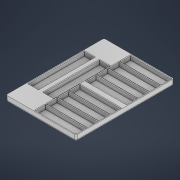
# Autodesk Inventor part: Pocker higher half
Saved by Autodesk Inventor 2022 (Build 260153000, 153)
## iProperties
Created: 2021-05-24
Part Number: Pocker higher half
Material: Aluminum 6061-AHC
Document SubType Name: Modeling
Designer: Albert L Tomberg
Density: 2.7 g/cm^3
Appearance: Aluminum - Polished
Author: Albert L Tomberg
Autodesk Inventor part; units mm, degrees
ref_plane "YZ Plane" through (0, 0, 0) normal (1, 0, 0) x (0, 1, 0)
ref_plane "XZ Plane" through (0, 0, 0) normal (0, 1, 0) x (-1, 0, 0)
ref_plane "XY Plane" through (0, 0, 0) normal (0, 0, 1) x (1, 0, 0)
sketch "Sketch1" plane through (0, 0, 0) normal (0, 1, 0) x (-1, 0, 0)
  line L0 (0, 0) -> (250, 0)
  line L1 (250, 0) -> (250, -350)
  line L2 (250, -350) -> (0, -350)
  line L3 (0, -350) -> (0, 0)
  dimension "d0" = 250
  dimension "d1" = 350
  constraints: 8 end point, 2 parallel, 1 horizontal, 1 perpendicular
  measures "d0" distance of L1.end L2.end
  measures "d1" distance of L0.end L1.end
extrude "Extrusion1" add sketch "Sketch1" along normal blind 20
sketch "Sketch2" plane through (0, 20, 0) normal (0, 1, 0) x (1, 0, 0)
  line L0 (-5, 5) -> (-150, 5)
  line L1 (-150, 5) -> (-150, 41)
  line L2 (-150, 41) -> (-5, 41)
  line L3 (-5, 41) -> (-5, 5)
  line L4 (-250, 0) -> (0, 0) projected
  line L5 (-250, 350) -> (-250, 0) projected
  line L6 (-150, 41) -> (-150, 46)
  line L7 (-150, 46) -> (-5, 46)
  line L8 (-5, 46) -> (-5, 82)
  line L9 (-5, 82) -> (-150, 82)
  line L10 (-150, 82) -> (-150, 46)
  line L11 (-150, 82) -> (-150, 87)
  line L12 (-150, 87) -> (-5, 87)
  line L13 (-5, 87) -> (-5, 123)
  line L14 (-5, 123) -> (-150, 123)
  line L15 (-150, 123) -> (-150, 87)
  line L16 (-150, 123) -> (-150, 128)
  line L17 (-150, 128) -> (-5, 128)
  line L18 (-5, 128) -> (-5, 164)
  line L19 (-5, 164) -> (-150, 164)
  line L20 (-150, 164) -> (-150, 128)
  line L21 (-5, 345) -> (-150, 345)
  line L22 (-150, 345) -> (-150, 309)
  line L23 (-150, 309) -> (-5, 309)
  line L24 (-5, 309) -> (-5, 345)
  line L25 (-5, 309) -> (-5, 304)
  line L26 (-5, 304) -> (-5, 268)
  line L27 (-5, 268) -> (-150, 268)
  line L28 (-150, 268) -> (-150, 304)
  line L29 (-150, 304) -> (-5, 304)
  line L30 (0, 0) -> (0, 350) projected
  line L31 (-150, 268) -> (-150, 263)
  line L32 (-150, 263) -> (-5, 263)
  line L33 (-5, 263) -> (-5, 227)
  line L34 (-5, 227) -> (-150, 227)
  line L35 (-150, 227) -> (-150, 263)
  line L36 (-5, 227) -> (-5, 222)
  line L37 (-5, 222) -> (-150, 222)
  line L38 (-150, 222) -> (-150, 186)
  line L39 (-150, 186) -> (-5, 186)
  line L40 (-5, 186) -> (-5, 222)
  line L41 (0, 350) -> (-250, 350) projected
  line L42 (-245, 75) -> (-245, 275)
  line L43 (-245, 275) -> (-209, 275)
  line L44 (-209, 275) -> (-209, 75)
  line L45 (-209, 75) -> (-245, 75)
  line L46 (-155, 75) -> (-155, 275)
  line L47 (-155, 275) -> (-191, 275)
  line L48 (-191, 275) -> (-191, 75)
  line L49 (-191, 75) -> (-155, 75)
  dimension "d4" = 145
  dimension "d5" = 36
  dimension "d6" = 5
  dimension "d7" = 100
  dimension "d8" = 5
  dimension "d9" = 36
  dimension "d10" = 5
  dimension "d11" = 36
  dimension "d12" = 5
  dimension "d13" = 36
  dimension "d14" = 36
  dimension "d15" = 5
  dimension "d16" = 36
  dimension "d17" = 5
  dimension "d18" = 36
  dimension "d19" = 5
  dimension "d20" = 36
  dimension "d21" = 5
  dimension "d22" = 5
  dimension "d23" = 5
  dimension "d24" = 200
  dimension "d25" = 36
  dimension "d26" = 36
  dimension "d27" = 5
  dimension "d28" = 75
  dimension "d29" = 18
  dimension "d30" = 75
  dimension "d31" = 75
  constraints: 92 end point, 25 perpendicular, 22 point on line, 6 parallel, 2 horizontal, 2 vertical
  measures "d4" distance of L1.end L2.end
  measures "d5" distance of L0.end L1.end
  measures "d6" distance between parallel lines of L4 L0
  measures "d7" distance between parallel lines of L5 L1
  measures "d8" distance of L1.end L6.end
  measures "d9" distance of L7.end L8.end
  measures "d10" distance of L9.end L11.end
  measures "d11" distance of L12.end L13.end
  measures "d12" distance of L14.end L16.end
  measures "d13" distance of L17.end L18.end
  measures "d14" distance of L21.end L22.end
  measures "d15" distance of L23.end L25.end
  measures "d16" distance of L25.end L26.end
  measures "d17" distance of L27.end L31.end
  measures "d18" distance of L32.end L33.end
  measures "d19" distance of L33.end L36.end
  measures "d20" distance of L37.end L38.end
  measures "d21" distance between parallel lines of L41 L21
  measures "d22" distance between parallel lines of L30 L8
  measures "d23" distance between parallel lines of L30 L13
  measures "d24" distance of L42.start L42.end
  measures "d25" distance of L42.end L43.end
  measures "d26" distance of L46.end L47.end
  measures "d27" distance between parallel lines of L5 L42
  measures "d28" distance between parallel lines of L4 L45
  measures "d29" distance between parallel lines of L44 L48
  measures "d30" distance between parallel lines of L4 L49
  measures "d31" distance between parallel lines of L41 L47
extrude "Extrusion2" cut sketch "Sketch2" against normal blind 15 contours L20 L19 L18 L17 | L15 L14 L13 L12 | L10 L9 L8 L7 | L0 L1 L2 L3 | L24 L23 L22 L21 | L40 L39 L38 L37 | L32 L33 L34 L35 | L26 L27 L28 L29 | L42 L43 L44 L45 | L49 L48 L47 L46
fillet "Fillet1" radius 5 8 edges at (-125, 0, 0) (0, 10, 0) (0, 0, -175) (0, 10, -350) (-125, 0, -350) (-250, 10, -350) (-250, 0, -175) (-250, 10, 0)
fillet "Fillet2" radius 1 79 edges at (-150, 5, -23) (-77.5, 5, -41) (-150, 12.5, -41) (-77.5, 5, -5) (-5, 5, -23) (-5, 5, -64) (-5, 5, -105) (-5, 5, -146) (-5, 5, -204) (-5, 5, -245) (-5, 5, -286) (-5, 12.5, -268) (-5, 12.5, -263) (-77.5, 5, -268) (-77.5, 5, -263) (-5, 12.5, -304) (-77.5, 5, -304) (-77.5, 5, -309) (-5, 12.5, -309) (-5, 5, -327) (-5, 12.5, -345) (-77.5, 5, -345) (-150, 12.5, -345) (-150, 5, -327) (-150, 12.5, -304) (-150, 12.5, -309) (-150, 12.5, -268) (-150, 12.5, -263) (-150, 5, -245) (-155, 5, -175) (-77.5, 5, -227) (-150, 12.5, -227) (-150, 12.5, -222) (-77.5, 5, -222) (-150, 5, -204) (-77.5, 5, -186) (-150, 12.5, -186) (-5, 12.5, -186) (-5, 12.5, -222) (-77.5, 5, -164) (-5, 12.5, -164) (-5, 12.5, -128) (-5, 12.5, -123) (-77.5, 5, -123) (-77.5, 5, -128) (-150, 12.5, -164) (-150, 12.5, -128) (-150, 12.5, -123) (-150, 12.5, -87) (-150, 5, -105) (-77.5, 5, -87) (-5, 12.5, -87) (-77.5, 5, -82) (-150, 5, -64) (-77.5, 5, -46) (-5, 12.5, -46) (-5, 12.5, -82) (-150, 12.5, -82) (-150, 12.5, -46) (-150, 12.5, -5) (-150, 5, -286) (-5, 12.5, -5) (-5, 12.5, -41) (-5, 12.5, -227) (-173, 5, -275) (-191, 5, -175) (-191, 12.5, -275) (-155, 12.5, -275) (-155, 12.5, -75) (-173, 5, -75) (-191, 12.5, -75) (-209, 12.5, -75) (-209, 5, -175) (-209, 12.5, -275) (-227, 5, -275) (-245, 5, -175) (-245, 12.5, -275) (-245, 12.5, -75) (-227, 5, -75)
fillet "Fillet3" radius 2 80 edges at (-5.2929, 20, -40.7071) (-5, 20, -23) (-5.2929, 20, -5.2929) (-77.5, 20, -5) (-149.7071, 20, -5.2929) (-150, 20, -23) (-149.7071, 20, -40.7071) (-77.5, 20, -41) (-149.7071, 20, -46.2929) (-150, 20, -64) (-149.7071, 20, -81.7071) (-77.5, 20, -82) (-5.2929, 20, -81.7071) (-5, 20, -64) (-5.2929, 20, -46.2929) (-77.5, 20, -46) (-149.7071, 20, -87.2929) (-150, 20, -105) (-149.7071, 20, -122.7071) (-77.5, 20, -123) (-5.2929, 20, -122.7071) (-5, 20, -105) (-5.2929, 20, -87.2929) (-77.5, 20, -87) (-149.7071, 20, -128.2929) (-150, 20, -146) (-149.7071, 20, -163.7071) (-77.5, 20, -164) (-5.2929, 20, -163.7071) (-5, 20, -146) (-5.2929, 20, -128.2929) (-77.5, 20, -128) (-149.7071, 20, -186.2929) (-150, 20, -204) (-149.7071, 20, -221.7071) (-77.5, 20, -222) (-5.2929, 20, -221.7071) (-5, 20, -204) (-5.2929, 20, -186.2929) (-77.5, 20, -186) (-149.7071, 20, -227.2929) (-150, 20, -245) (-149.7071, 20, -262.7071) (-77.5, 20, -263) (-5.2929, 20, -262.7071) (-5, 20, -245) (-5.2929, 20, -227.2929) (-77.5, 20, -227) (-149.7071, 20, -268.2929) (-150, 20, -286) (-149.7071, 20, -303.7071) (-77.5, 20, -304) (-5.2929, 20, -303.7071) (-5, 20, -286) (-5.2929, 20, -268.2929) (-77.5, 20, -268) (-149.7071, 20, -309.2929) (-150, 20, -327) (-149.7071, 20, -344.7071) (-77.5, 20, -345) (-5.2929, 20, -344.7071) (-5, 20, -327) (-5.2929, 20, -309.2929) (-77.5, 20, -309) (-155.2929, 20, -75.2929) (-173, 20, -75) (-190.7071, 20, -75.2929) (-191, 20, -175) (-190.7071, 20, -274.7071) (-173, 20, -275) (-155.2929, 20, -274.7071) (-155, 20, -175) (-209.2929, 20, -75.2929) (-227, 20, -75) (-244.7071, 20, -75.2929) (-245, 20, -175) (-244.7071, 20, -274.7071) (-227, 20, -275) (-209.2929, 20, -274.7071) (-209, 20, -175)
body "Solid1"
